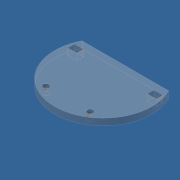
# Autodesk Inventor part: S1702_couverclebas
Saved by Autodesk Inventor 2015 SP2 (Build 190223200, 223)
## iProperties
Created: 2017-10-30
Part Number: S1702_couverclebas
Project: S1702_Circuit_Course
Material: Plastique PMMA
Description: Couvercle Bas
Document SubType Name: Modeling
Designer: Benoit.CURCHOD2
Authority: Ø44x3
Density: 1.188 g/cm^3
Appearance: Transparent - Clair
Mass: 3.31821 g
Surface Area: 26.0683 cm^2
Volume: 2.79311 cm^3
Material number: ---
Author: Benoit.CURCHOD2
Autodesk Inventor part; units mm, degrees
ref_plane "Plan YZ" through (0, 0, 0) normal (1, 0, 0) x (0, 1, 0)
ref_plane "Plan XZ" through (0, 0, 0) normal (0, 1, 0) x (-1, 0, 0)
ref_plane "Plan XY" through (0, 0, 0) normal (0, 0, 1) x (1, 0, 0)
sketch "Esquisse1" plane through (0, 0, 0) normal (0, 0, 1) x (1, 0, 0)
  line L0 (19.5959, 10) -> (-19.5959, 10)
  line L1 (19.5959, 10) -> (-19.5959, 10) construction
  line L2 (-20, 7) -> (-16, 7)
  line L3 (-16, 7) -> (-16, 4)
  line L4 (-16, 4) -> (-20, 4)
  line L5 (-20, 4) -> (-20, 7)
  line L6 (20, 7) -> (16, 7)
  line L7 (16, 7) -> (16, 4)
  line L8 (16, 4) -> (20, 4)
  line L9 (20, 4) -> (20, 7)
  line L10 (0, -28.4) -> (0, 16.4) construction
  line L11 (-30.8, 0) -> (30.8, 0) construction
  arc A0 (-19.5959, 10) -> (19.5959, 10) centre (0, 0) ccw
  dimension "d61" = 4
  dimension "d63" = 3
  dimension "d68" = 4
  dimension "d69" = 16
  dimension "d70" = 10
  dimension "d89" = 22
  constraints: 20 end point, 2 collinear, 2 horizontal, 2 parallel, 2 point on circle, 1 centre point, 1 coincident, 1 perpendicular, 2 other
  measures "d61" distance between parallel lines of L3 L5
  measures "d63" distance between parallel lines of L4 L2
  measures "d68" distance between parallel lines of L11 L4
  measures "d69" distance between parallel lines of L10 L3
  measures "d70" distance between parallel lines of L11 L0
  measures "d89" radius of A0
extrude "Extrusion5" add sketch "Esquisse1" along normal blind 3
sketch "Esquisse13" plane through (0, 0, 0) normal (0, 0, -1) x (-1, 0, 0)
  line L0 (30.8, 0) -> (-30.8, 0) construction
  line L1 (0, -28.4) -> (0, 16.4) construction
  arc A0 (-18.8, 0) -> (18.8, 0) centre (0, 0) ccw construction
  point P0 (-10, -15.9198)
  point P1 (10, -15.9198)
  dimension "d79" = 20
  dimension "d87" = 18.8
  constraints: 3 point on circle, 2 point on line, 1 centre point, 1 coincident, 1 symmetric about line
  measures "d79" distance of point (10, -15.92) point (-10, -15.92)
  measures "d87" radius of A0
hole "Perçage4" at (10, -15.9198, 0) at (-10, -15.9198, 0) direction (0, 0, 1) diameter 2.459 end through all thread size "M3x0.5" class "6H" standard "ISO M"
